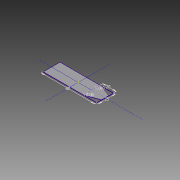
# Autodesk Inventor part: BandBack
Saved by Autodesk Inventor 2016 (Build 200138000, 138)
## iProperties
Created: 2015-04-10
Part Number: BandBack
Material: Generic
Document SubType Name: Modeling
Designer: Erin
Density: 1 g/cm^3
Appearance: Default
Author: Erin
Autodesk Inventor part; units mm, degrees
ref_plane "YZ Plane" through (0, 0, 0) normal (1, 0, 0) x (0, 1, 0)
ref_plane "XZ Plane" through (0, 0, 0) normal (0, 1, 0) x (-1, 0, 0)
ref_plane "XY Plane" through (0, 0, 0) normal (0, 0, 1) x (1, 0, 0)
sketch "Sketch1" plane through (0, 0, 0) normal (0, 0, 1) x (1, 0, 0)
  line L0 (-40, 12.5) -> (40, 12.5)
  line L1 (40, 12.5) -> (40, -12.5)
  line L2 (40, -12.5) -> (-40, -12.5)
  line L3 (-40, -12.5) -> (-40, 12.5)
  line L4 (-58.4065, 0) -> (96.114, 0) construction
  line L5 (0, 47.121) -> (0, -49.5625) construction
  line L6 (20, 12.5) -> (20, -12.5)
  line L7 (20, 12.5) -> (40, 5.2206)
  line L8 (20, -12.5) -> (40, -5.2206)
  point P0 (0, 0)
  point P1 (0, 12.5)
  point P2 (40, 0)
  dimension "d0" = 80
  dimension "d1" = 25
  dimension "d11" = 20
  dimension "d16" = 70
  dimension "d17" = 70
  constraints: 18 end point, 4 perpendicular, 4 point on line, 2 horizontal, 2 midpoint, 2 parallel, 1 horizontal alignment, 1 vertical, 1 vertical alignment
  measures "d0" distance of L1.end L2.end
  measures "d1" distance of L0.end L1.end
  measures "d11" distance between parallel lines of L6 L1
  measures "d16" angle of L6 L7
  measures "d17" angle of L6 L8
extrude "Extrusion4" add sketch "Sketch1" along normal blind 0.2 contours L0 L6 L2 L3 | L7 L1 L8 L6
extrude "Extrusion5" add sketch "Sketch1" along normal blind 0.4 contours L7 L1 L8 L6
equation "\"d18\" = material"
equation "\"d20\" = 2 * material"
equation "\"material\" = 0.2"
body "Solid2"
